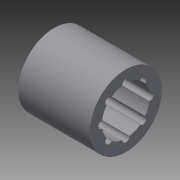
# Autodesk Inventor part: Part3
Saved by Autodesk Inventor 2015 (Build 190159000, 159)
## iProperties
Created: 2015-03-02
Part Number: Part3
Material: Generic
Document SubType Name: Modeling
Designer: WASHHSST
Density: 1 g/cm^3
Appearance: Default
Author: WASHHSST
Autodesk Inventor part; units mm, degrees
ref_plane "YZ Plane" through (0, 0, 0) normal (1, 0, 0) x (0, 1, 0)
ref_plane "XZ Plane" through (0, 0, 0) normal (0, 1, 0) x (-1, 0, 0)
ref_plane "XY Plane" through (0, 0, 0) normal (0, 0, 1) x (1, 0, 0)
sketch "Sketch1" plane through (0, 0, 0) normal (1, 0, 0) x (0, 1, 0)
  circle A0 centre (0, 0) radius 38.1
  dimension "d0" = 76.2
  constraints: 1 centre point, 1 coincident
  measures "d0" diameter of A0
extrude "Extrusion1" add sketch "Sketch1" along normal blind 76.2
sketch "Sketch2" plane through (76.2, 0, 0) normal (1, 0, 0) x (0, 0, -1)
  circle A0 centre (0, 0) radius 25.4
  dimension "d3" = 50.8
  constraints: 1 centre point, 1 coincident
  measures "d3" diameter of A0
extrude "Extrusion2" cut sketch "Sketch2" against normal blind 152.4
sketch "Sketch3" plane through (76.2, 0, 0) normal (1, 0, 0) x (0, 0, -1)
  circle A0 centre (0, 0) radius 25.4
  circle A1 centre (0, 0) radius 25.4 projected
  circle A2 centre (0.0066, 25.4) radius 3.81
  circle A3 centre (-17.9558, 17.9652) radius 3.81
  circle A4 centre (-25.4, 0.0066) radius 3.81
  circle A5 centre (-17.9652, -17.9558) radius 3.81
  circle A6 centre (-0.0066, -25.4) radius 3.81
  circle A7 centre (17.9558, -17.9652) radius 3.81
  circle A8 centre (25.4, -0.0066) radius 3.81
  circle A9 centre (17.9652, 17.9558) radius 3.81
  dimension "d6" = 7.62
  dimension "d9" = 360
  constraints: 8 centre point, 1 coincident, 22 other
  measures "d6" diameter of A2
extrude "Extrusion3" cut sketch "Sketch3" against normal blind 152.4 contours A0 A8 | A0 A8 | A9 A0 | A0 A9 | A7 A0 | A0 A7 | A2 A0 | A0 A2 | A6 A0 | A0 A6 | A3 A0 | A0 A3 | A5 A0 | A0 A5 | A4 A0 | A0 A4
body "Solid1"
